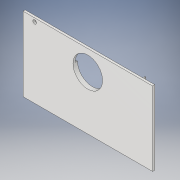
# Autodesk Inventor part: base
Saved by Autodesk Inventor 2019 (Build 230136000, 136)
## iProperties
Created: 2020-03-02
Part Number: base
Material: Acetal Resin, White
Document SubType Name: Sheet Metal
Designer: PRAVEEN
Density: 1.425 g/cm^3
Sheet Metal Rule: Default_mm
Appearance: Smooth - White
Author: PRAVEEN
Autodesk Inventor part; units mm, degrees
ref_plane "YZ Plane" through (0, 0, 0) normal (1, 0, 0) x (0, 1, 0)
ref_plane "XZ Plane" through (0, 0, 0) normal (0, 1, 0) x (-1, 0, 0)
ref_plane "XY Plane" through (0, 0, 0) normal (0, 0, 1) x (1, 0, 0)
sketch "Sketch1" plane through (0, 0, 0) normal (0, 0, 1) x (1, 0, 0)
  line L0 (0, 0) -> (700, 0)
  line L1 (700, 0) -> (700, -400)
  line L2 (700, -400) -> (0, -400)
  line L3 (0, -400) -> (0, 0)
  dimension "d0" = 700
  dimension "d1" = 400
  constraints: 8 end point, 2 parallel, 1 horizontal, 1 perpendicular
  measures "d0" distance of L1.end L2.end
  measures "d1" distance of L0.end L1.end
extrude "Extrusion1" add sketch "Sketch1" along normal blind 12
sketch "Sketch2" plane through (0, 0, 0) normal (0, 0, -1) x (-1, 0, 0)
  circle A0 centre (-350, -200) radius 80
  point P0 (0, 0)
  dimension "d4" = 160
  constraints: 1 centre point
  measures "d4" diameter of A0
extrude "Extrusion2" cut sketch "Sketch2" against normal blind 12
sketch "Sketch3" plane through (0, 0, 0) normal (0, 0, -1) x (-1, 0, 0)
  arc A0 (-430, -200) -> (-270, -200) centre (-350, -200) ccw
  line L0 (-270, -200) -> (-270, 0)
  line L1 (-430, -200) -> (-430, 0)
  line L2 (-265, 0) -> (-265, -200)
  arc A1 (-435, -200) -> (-265, -200) centre (-350, -200) ccw
  line L3 (-435, -200) -> (-435, 0)
  line L4 (-65, 0) -> (-65, -200)
  arc A2 (-635, -200) -> (-65, -200) centre (-350, -200) ccw
  line L5 (-635, -200) -> (-635, 0)
  line L6 (-60, 0) -> (-60, -200)
  arc A3 (-640, -200) -> (-60, -200) centre (-350, -200) ccw
  line L7 (-640, -200) -> (-640, 0)
  line L8 (-60, 0) -> (-65, 0)
  line L9 (-700, 0) -> (0, 0) projected
  line L10 (-430, 0) -> (-435, 0)
  line L11 (-635, 0) -> (-640, 0)
  line L12 (-265, 0) -> (-270, 0)
  dimension "d7" = 5
  dimension "d8" = 200
  dimension "d9" = 5
  constraints: 24 end point, 8 point on circle, 4 centre point, 3 collinear, 2 vertical, 1 coincident, 1 horizontal, 1 tangent, 7 other
  measures "d7" distance between parallel lines of L0 L2
  measures "d8" radial gap between concentric circles of A1 A2
  measures "d9" radial gap between concentric circles of A2 A3
extrude "Extrusion3" add sketch "Sketch3" along normal blind 12 contours A0 L0 L9 L2 A1 L3 L1 | L5 A2 L4 L8 L6 A3 L7 L9
sketch "Sketch4" plane through (700, -400, 0) normal (1, 0, 0) x (0, 0, -1)
  line L0 (0, 0) -> (-12, 0) projected
  line L1 (0, 0) -> (-12, 0)
  line L2 (-12, 0) -> (-12, -90)
  line L3 (-12, -90) -> (0, -90)
  line L4 (0, -90) -> (0, 0)
  point P0 (0, 400)
  dimension "d12" = 90
  constraints: 8 end point, 2 parallel, 1 horizontal, 1 perpendicular
  measures "d12" distance of L2.end L1.end
extrude "Extrusion4" add sketch "Sketch4" against normal blind 700
sketch "Sketch5" plane through (700, 0, 12) normal (1, 0, 0) x (0, 0, -1)
  line L0 (12, 0) -> (0, 0) projected
  line L1 (0, 0) -> (88.8281, 0)
  line L2 (88.8281, 0) -> (88.8281, -90)
  line L3 (88.8281, -90) -> (0, -90)
  line L4 (0, -90) -> (0, 0)
  dimension "d15" = 90
  constraints: 8 end point, 2 parallel, 1 horizontal, 1 perpendicular
  measures "d15" distance of L1.end L2.end
extrude "Extrusion5" cut sketch "Sketch5" against normal blind 10000
sketch "Sketch6" plane through (0, -490, 0) normal (-1, 0, 0) x (0, 0, 1)
  line L0 (0, 290) -> (0, 400) projected
  line L1 (0, 400) -> (-31.175, 400)
  line L2 (-31.175, 400) -> (-31.175, 290)
  line L3 (-31.175, 290) -> (0, 290)
  line L4 (0, 290) -> (0, 400)
  point P0 (0, 490)
  constraints: 8 end point, 2 parallel, 1 horizontal, 1 perpendicular
extrude "Extrusion6" cut sketch "Sketch6" against normal blind 500
sketch "Sketch7" plane through (0, 0, 0) normal (0, 0, -1) x (-1, 0, 0)
  circle A0 centre (-52.4557, -179.1018) radius 2.5
  circle A1 centre (-52.4557, -169.2668) radius 2.5
  point P0 (0, 0)
  dimension "d20" = 5
  dimension "d21" = 5
  constraints: 2 centre point
  measures "d20" diameter of A0
  measures "d21" diameter of A1
extrude "Extrusion7" add sketch "Sketch7" along normal blind 7
fillet "Fillet1" radius 2.5 2 edges at (54.9557, -169.2668, -7) (54.9557, -179.1018, -7)
fillet "Fillet2" radius 0.1 2 edges at (54.9557, -169.2668, 0) (54.9557, -179.1018, 0)
sketch "Sketch8" plane through (0, 0, 0) normal (0, 0, -1) x (-1, 0, 0)
  circle A0 centre (-63.0207, -108.7531) radius 10
  point P0 (0, 0)
  dimension "d26" = 20
  constraints: 1 centre point
  measures "d26" diameter of A0
extrude "Extrusion8" cut sketch "Sketch8" against normal blind 20
equation "\"BendRadius\" = Thickness"
equation "\"BendReliefWidth\" = Thickness"
equation "\"BendReliefDepth\" = 0.5 * Thickness"
equation "\"CornerReliefSize\" = 4 * Thickness"
equation "\"MinimumRemnant\" = 2 * Thickness"
equation "\"TransitionRadius\" = BendRadius"
equation "\"JacobiRadiusSize\" = BendRadius"
equation "\"GapSize\" = Thickness"
equation "\"Thickness\" = 0.5"
body "Solid1"
